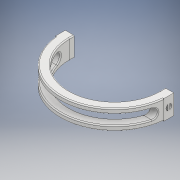
# Autodesk Inventor part: BottomCircleArm
Saved by Autodesk Inventor 2017 (Build 210142000, 142)
## iProperties
Created: 2017-02-18
Part Number: BottomCircleArm
Material: ABS Plastic
Document SubType Name: Modeling
Designer: aribu
Density: 1.06 g/cm^3
Appearance: Smooth - White
Author: aribu
Autodesk Inventor part; units mm, degrees
ref_plane "YZ Plane" through (0, 0, 0) normal (1, 0, 0) x (0, 1, 0)
ref_plane "XZ Plane" through (0, 0, 0) normal (0, 1, 0) x (-1, 0, 0)
ref_plane "XY Plane" through (0, 0, 0) normal (0, 0, 1) x (1, 0, 0)
sketch "Sketch1" plane through (0, 0, 0) normal (0, 0, 1) x (1, 0, 0)
  arc A0 (-46, 0) -> (46, 0) centre (0, 0) ccw
  arc A1 (-54.7723, -5) -> (54.7723, -5) centre (0, 0) ccw
  line L0 (-55, 0) -> (-55, 0)
  line L1 (50, 0) -> (50, 0)
  line L2 (-46, 5) -> (-55, 5)
  line L3 (-55, 5) -> (-55, -5)
  line L4 (-55, -5) -> (-54.7723, -5)
  line L5 (-46, 0) -> (-46, 5)
  line L6 (46, 5) -> (55, 5)
  line L7 (55, 5) -> (55, -5)
  line L8 (55, -5) -> (54.7723, -5)
  line L9 (46, 0) -> (46, 5)
  dimension "d0" = 92
  dimension "d1" = 110
  dimension "d26" = 9
  dimension "d27" = 10
  dimension "d28" = 5
  dimension "d29" = 9
  dimension "d30" = 10
  dimension "d32" = 5
  constraints: 20 end point, 4 parallel, 4 point on circle, 2 centre point, 2 coincident, 2 horizontal, 2 perpendicular
  measures "d0" diameter of A0
  measures "d1" diameter of A1
  measures "d26" distance of L2.start L2.end
  measures "d27" distance of L2.end L3.end
  measures "d28" distance from line of L2 L0.end
  measures "d29" distance of L6.start L6.end
  measures "d30" distance of L6.end L7.end
  measures "d32" distance from line of L5.start L6
extrude "Extrusion1" add sketch "Sketch1" along normal blind 20
sketch "Sketch2" plane through (55, -5, 0) normal (1, 0, 0) x (0, 0, -1)
  arc A0 (-5, -10) -> (-15, -10) centre (-10, -10) ccw
  line L0 (0, 10) -> (0, 0)
  line L1 (0, 0) -> (-10, 0)
  line L2 (-15, -10) -> (-15, -70)
  line L3 (-15, -70) -> (-5, -70)
  line L4 (-5, -70) -> (-5, -10)
  line L5 (0, 0) -> (-10, 0)
  line L6 (0, 10) -> (0, 0)
  line L7 (0, 0) -> (0, 10) projected
  dimension "d6" = 10
  dimension "d7" = 10
  dimension "d8" = 10
  dimension "d14" = 60
  dimension "d15" = 0
  dimension "d16" = 0
  dimension "d17" = 10
  dimension "d37" = 0
  constraints: 14 end point, 2 point on circle, 2 tangent, 1 centre point, 1 perpendicular, 1 vertical
  measures "d6" diameter of A0
  measures "d7" distance from line of L0 A0.centre
  measures "d8" distance from line of L1 A0.centre
  measures "d14" distance of L2.start L2.end
  measures "d15" distance between parallel lines of L5 L1
  measures "d16" distance between parallel lines of L6 L0
  measures "d17" distance of L2.end L3.end
  measures "d37" distance between parallel lines of L7 L0
extrude "Extrusion2" cut sketch "Sketch2" against normal blind 120
fillet "Fillet1" radius 1 12 edges at (44.8999, -10, 9.9957) (0, -46, 15) (-44.8999, -10, 9.9957) (0, -46, 5) (-54.0833, -10, 9.9953) (0, -55, 15) (54.0833, -10, 9.9953) (0, -55, 5) (0, -55, 20) (0, -55, 0) (0, -46, 0) (0, -46, 20)
sketch "Sketch3" plane through (55, -5, 0) normal (1, 0, 0) x (0, 0, -1)
  line L0 (-12.7753, 4) -> (-7.2247, 4)
  line L1 (-7.2247, 6) -> (-12.7753, 6)
  arc A0 (-12.7753, 4) -> (-7.2247, 4) centre (-10, 5) ccw
  arc A1 (-7.2247, 6) -> (-12.7753, 6) centre (-10, 5) ccw
  line L2 (-20, 0) -> (-20, 10) projected
  point P0 (1, 0)
  dimension "d33" = 10
  dimension "d34" = 2.95
  dimension "d35" = 2.95
  dimension "d36" = 2
  constraints: 4 end point, 4 point on circle, 2 centre point, 1 horizontal, 1 parallel
  measures "d33" distance from line of L2 A0.centre
  measures "d34" radius of A1
  measures "d35" radius of A0
  measures "d36" distance between parallel lines of L1 L0
extrude "Extrusion3" cut sketch "Sketch3" against normal blind 10
equation "\"d28\" = 0.5 * d27"
equation "\"d30\" = d27"
body "Solid1"
